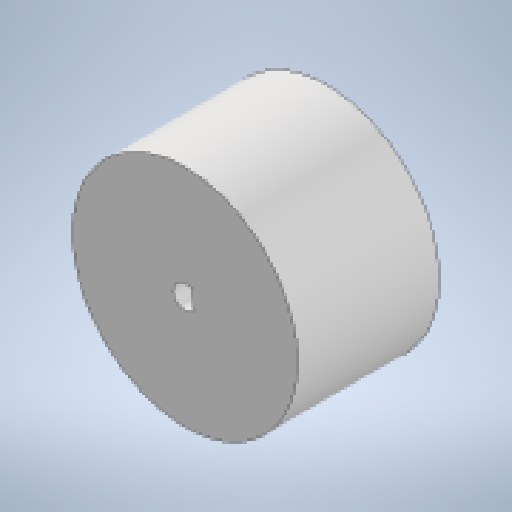
# Autodesk Inventor part: opona_nowa
Saved by Autodesk Inventor 2023 (Build 270158000, 158)
## iProperties
Created: 2023-04-06
Part Number: opona_nowa
Material: Ogólny
Document SubType Name: Modeling
Designer: Kamil
Density: 1 g/cm^3
Appearance: Domyślna
Author: Kamil
Autodesk Inventor part; units mm, degrees
ref_plane "YZ Plane" through (0, 0, 0) normal (1, 0, 0) x (0, 1, 0)
ref_plane "XZ Plane" through (0, 0, 0) normal (0, 1, 0) x (-1, 0, 0)
sketch "Szkic1" plane through (0, 0, 0) normal (0, 0, 1) x (1, 0, 0)
  circle A0 centre (0, 0) radius 14.5
  arc A1 (0.8877, 1.2091) -> (1.103, -1.0166) centre (0, 0) ccw projected
  line L0 (0.8877, 1.2091) -> (1.103, -1.0166) projected
  dimension "d0" = 29
  constraints: 1 centre point, 1 coincident
  measures "d0" diameter of A0
ref_plane "Płaszczyzna konstrukcyjna1" through (-9.6084, -5, 18.3) normal (0, 0, 1) x (1, 0, 0)
extrude "Wyciągnięcie proste1" add sketch "Szkic1" along normal up to surface (18.3 mm away)
